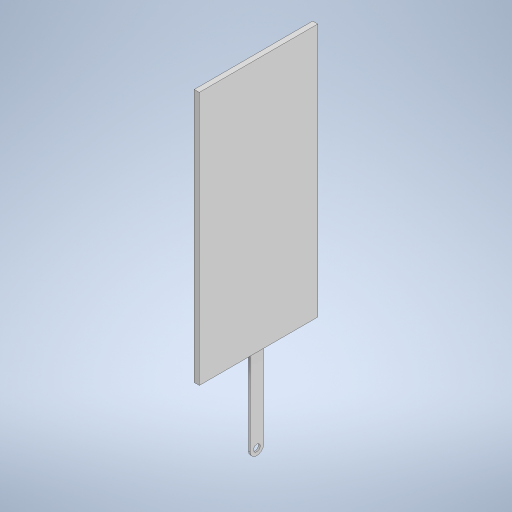
# Autodesk Inventor part: reka
Saved by Autodesk Inventor 2023 (Build 270158000, 158)
## iProperties
Created: 2023-07-08
Part Number: reka
Material: Ogólny
Document SubType Name: Modeling
Designer: Kamil
Density: 1 g/cm^3
Appearance: Domyślna
Author: Kamil
Autodesk Inventor part; units mm, degrees
ref_plane "YZ Plane" through (0, 0, 0) normal (1, 0, 0) x (0, 1, 0)
ref_plane "XZ Plane" through (0, 0, 0) normal (0, 1, 0) x (-1, 0, 0)
ref_plane "XY Plane" through (0, 0, 0) normal (0, 0, 1) x (1, 0, 0)
sketch "Szkic1" plane through (0, 0, 0) normal (1, 0, 0) x (0, 1, 0)
  circle A0 centre (0, 0) radius 4
  circle A1 centre (0, 0) radius 2
  line L0 (0, 4) -> (200, 4)
  line L1 (200, 4) -> (200, -4)
  line L2 (200, -4) -> (0, -4)
  line L3 (0, -4) -> (0, 4)
  point P0 (0, -4)
  dimension "d0" = 8
  dimension "d1" = 4
  dimension "d2" = 200
  dimension "d3" = 8
  constraints: 8 end point, 2 coincident, 2 parallel, 1 centre point, 1 horizontal, 1 perpendicular, 3 other
  measures "d1" diameter of A1
  measures "d2" distance of L1.end L2.end
  measures "d3" distance of L0.end L1.end
extrude "Wyciągnięcie proste1" add sketch "Szkic1" along normal blind 1 contours A0 L3 A1 | A0 L0 L1 L2 | L3 A1 A0
sketch "Szkic2" plane through (1, 0, 0) normal (1, 0, 0) x (0, 0, -1)
  line L0 (-35, 200) -> (35, 200)
  line L1 (35, 200) -> (35, 50)
  line L2 (35, 50) -> (-35, 50)
  line L3 (-35, 50) -> (-35, 200)
  line L4 (4, 200) -> (-4, 200) projected
  point P0 (0, 0)
  point P1 (0, 200)
  point P2 (0, 200)
  point P3 (0, 200)
  dimension "d6" = 70
  dimension "d7" = 150
  constraints: 8 end point, 3 midpoint, 2 parallel, 1 coincident, 1 horizontal, 1 horizontal alignment, 1 perpendicular
  measures "d6" distance of L1.end L2.end
  measures "d7" distance of L0.end L1.end
extrude "Wyciągnięcie proste2" add sketch "Szkic2" along normal blind 1 and the other way blind 2
